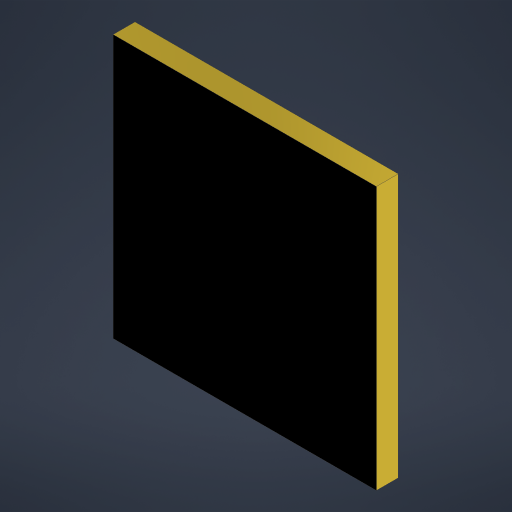
# Autodesk Inventor part: šachovnice
Saved by Autodesk Inventor 2023 (Build 270158000, 158)
## iProperties
Created: 2023-04-20
Part Number: šachovnice
Material: Generic
Document SubType Name: Modeling
Designer: 19LBoreckyP
Density: 1 g/cm^3
Appearance: Wood - Painted White
Author: 19LBoreckyP
Autodesk Inventor part; units mm, degrees
(part 1 of 2)
ref_plane "YZ Plane" through (0, 0, 0) normal (1, 0, 0) x (0, 1, 0)
ref_plane "XZ Plane" through (0, 0, 0) normal (0, 1, 0) x (-1, 0, 0)
ref_plane "XY Plane" through (0, 0, 0) normal (0, 0, 1) x (1, 0, 0)
sketch "Sketch1" plane through (0, 0, 0) normal (0, 0, 1) x (1, 0, 0)
  line L0 (-28.2811, -25.3359) -> (21.7189, -25.3359)
  line L1 (21.7189, -25.3359) -> (21.7189, 24.6641)
  line L2 (21.7189, 24.6641) -> (-28.2811, 24.6641)
  line L3 (-28.2811, 24.6641) -> (-28.2811, -25.3359)
  line L4 (-28.2811, -25.3359) -> (21.7189, 24.6641) construction
  line L5 (21.7189, -25.3359) -> (-28.2811, 24.6641) construction
  line L6 (21.7189, 24.6641) -> (21.7189, 74.6641)
  line L7 (21.7189, 74.6641) -> (-28.2811, 74.6641)
  line L8 (-28.2811, 74.6641) -> (-28.2811, 24.6641)
  line L9 (-28.2811, 24.6641) -> (21.7189, 24.6641)
  line L10 (21.7189, 74.6641) -> (21.7189, 124.6641)
  line L11 (21.7189, 124.6641) -> (-28.2811, 124.6641)
  line L12 (-28.2811, 124.6641) -> (-28.2811, 74.6641)
  line L13 (-28.2811, 74.6641) -> (21.7189, 74.6641)
  line L14 (21.7189, 124.6641) -> (21.7189, 174.6641)
  line L15 (21.7189, 174.6641) -> (-28.2811, 174.6641)
  line L16 (-28.2811, 174.6641) -> (-28.2811, 124.6641)
  line L17 (-28.2811, 124.6641) -> (21.7189, 124.6641)
  line L18 (21.7189, 174.6641) -> (21.7189, 224.6641)
  line L19 (21.7189, 224.6641) -> (-28.2811, 224.6641)
  line L20 (-28.2811, 224.6641) -> (-28.2811, 174.6641)
  line L21 (-28.2811, 174.6641) -> (21.7189, 174.6641)
  line L22 (21.7189, 224.6641) -> (21.7189, 274.6641)
  line L23 (21.7189, 274.6641) -> (-28.2811, 274.6641)
  line L24 (-28.2811, 274.6641) -> (-28.2811, 224.6641)
  line L25 (-28.2811, 224.6641) -> (21.7189, 224.6641)
  line L26 (21.7189, 274.6641) -> (21.7189, 324.6641)
  line L27 (21.7189, 324.6641) -> (-28.2811, 324.6641)
  line L28 (-28.2811, 324.6641) -> (-28.2811, 274.6641)
  line L29 (-28.2811, 274.6641) -> (21.7189, 274.6641)
  line L30 (21.7189, 324.6641) -> (21.7189, 374.6641)
  line L31 (21.7189, 374.6641) -> (-28.2811, 374.6641)
  line L32 (-28.2811, 374.6641) -> (-28.2811, 324.6641)
  line L33 (-28.2811, 324.6641) -> (21.7189, 324.6641)
  line L34 (71.7189, -25.3359) -> (71.7189, 24.6641)
  line L35 (71.7189, 24.6641) -> (21.7189, 24.6641)
  line L36 (21.7189, 24.6641) -> (21.7189, -25.3359)
  line L37 (21.7189, -25.3359) -> (71.7189, -25.3359)
  line L38 (71.7189, 24.6641) -> (71.7189, 74.6641)
  line L39 (71.7189, 74.6641) -> (21.7189, 74.6641)
  line L40 (21.7189, 74.6641) -> (21.7189, 24.6641)
  line L41 (21.7189, 24.6641) -> (71.7189, 24.6641)
  line L42 (71.7189, 74.6641) -> (71.7189, 124.6641)
  line L43 (71.7189, 124.6641) -> (21.7189, 124.6641)
  line L44 (21.7189, 124.6641) -> (21.7189, 74.6641)
  line L45 (21.7189, 74.6641) -> (71.7189, 74.6641)
  line L46 (71.7189, 124.6641) -> (71.7189, 174.6641)
  line L47 (71.7189, 174.6641) -> (21.7189, 174.6641)
  line L48 (21.7189, 174.6641) -> (21.7189, 124.6641)
  line L49 (21.7189, 124.6641) -> (71.7189, 124.6641)
  line L50 (71.7189, 174.6641) -> (71.7189, 224.6641)
  line L51 (71.7189, 224.6641) -> (21.7189, 224.6641)
  line L52 (21.7189, 224.6641) -> (21.7189, 174.6641)
  line L53 (21.7189, 174.6641) -> (71.7189, 174.6641)
  line L54 (71.7189, 224.6641) -> (71.7189, 274.6641)
  line L55 (71.7189, 274.6641) -> (21.7189, 274.6641)
  line L56 (21.7189, 274.6641) -> (21.7189, 224.6641)
  line L57 (21.7189, 224.6641) -> (71.7189, 224.6641)
  line L58 (71.7189, 274.6641) -> (71.7189, 324.6641)
  line L59 (71.7189, 324.6641) -> (21.7189, 324.6641)
  line L60 (21.7189, 324.6641) -> (21.7189, 274.6641)
  line L61 (21.7189, 274.6641) -> (71.7189, 274.6641)
  line L62 (71.7189, 324.6641) -> (71.7189, 374.6641)
  line L63 (71.7189, 374.6641) -> (21.7189, 374.6641)
  line L64 (21.7189, 374.6641) -> (21.7189, 324.6641)
  line L65 (21.7189, 324.6641) -> (71.7189, 324.6641)
  line L66 (121.7189, -25.3359) -> (121.7189, 24.6641)
  line L67 (121.7189, 24.6641) -> (71.7189, 24.6641)
  line L68 (71.7189, 24.6641) -> (71.7189, -25.3359)
  line L69 (71.7189, -25.3359) -> (121.7189, -25.3359)
  line L70 (121.7189, 24.6641) -> (121.7189, 74.6641)
  line L71 (121.7189, 74.6641) -> (71.7189, 74.6641)
  line L72 (71.7189, 74.6641) -> (71.7189, 24.6641)
  line L73 (71.7189, 24.6641) -> (121.7189, 24.6641)
  line L74 (121.7189, 74.6641) -> (121.7189, 124.6641)
  line L75 (121.7189, 124.6641) -> (71.7189, 124.6641)
  line L76 (71.7189, 124.6641) -> (71.7189, 74.6641)
  line L77 (71.7189, 74.6641) -> (121.7189, 74.6641)
  line L78 (121.7189, 124.6641) -> (121.7189, 174.6641)
  line L79 (121.7189, 174.6641) -> (71.7189, 174.6641)
  line L80 (71.7189, 174.6641) -> (71.7189, 124.6641)
  line L81 (71.7189, 124.6641) -> (121.7189, 124.6641)
  line L82 (121.7189, 174.6641) -> (121.7189, 224.6641)
  line L83 (121.7189, 224.6641) -> (71.7189, 224.6641)
  line L84 (71.7189, 224.6641) -> (71.7189, 174.6641)
  line L85 (71.7189, 174.6641) -> (121.7189, 174.6641)
  line L86 (121.7189, 224.6641) -> (121.7189, 274.6641)
  line L87 (121.7189, 274.6641) -> (71.7189, 274.6641)
  line L88 (71.7189, 274.6641) -> (71.7189, 224.6641)
  line L89 (71.7189, 224.6641) -> (121.7189, 224.6641)
  line L90 (121.7189, 274.6641) -> (121.7189, 324.6641)
  line L91 (121.7189, 324.6641) -> (71.7189, 324.6641)
  line L92 (71.7189, 324.6641) -> (71.7189, 274.6641)
  line L93 (71.7189, 274.6641) -> (121.7189, 274.6641)
  line L94 (121.7189, 324.6641) -> (121.7189, 374.6641)
  line L95 (121.7189, 374.6641) -> (71.7189, 374.6641)
  line L96 (71.7189, 374.6641) -> (71.7189, 324.6641)
  line L97 (71.7189, 324.6641) -> (121.7189, 324.6641)
  line L98 (171.7189, -25.3359) -> (171.7189, 24.6641)
  line L99 (171.7189, 24.6641) -> (121.7189, 24.6641)
  line L100 (121.7189, 24.6641) -> (121.7189, -25.3359)
  line L101 (121.7189, -25.3359) -> (171.7189, -25.3359)
  line L102 (171.7189, 24.6641) -> (171.7189, 74.6641)
  line L103 (171.7189, 74.6641) -> (121.7189, 74.6641)
  line L104 (121.7189, 74.6641) -> (121.7189, 24.6641)
  line L105 (121.7189, 24.6641) -> (171.7189, 24.6641)
  line L106 (171.7189, 74.6641) -> (171.7189, 124.6641)
  line L107 (171.7189, 124.6641) -> (121.7189, 124.6641)
  line L108 (121.7189, 124.6641) -> (121.7189, 74.6641)
  line L109 (121.7189, 74.6641) -> (171.7189, 74.6641)
  line L110 (171.7189, 124.6641) -> (171.7189, 174.6641)
  line L111 (171.7189, 174.6641) -> (121.7189, 174.6641)
  line L112 (121.7189, 174.6641) -> (121.7189, 124.6641)
  line L113 (121.7189, 124.6641) -> (171.7189, 124.6641)
  line L114 (171.7189, 174.6641) -> (171.7189, 224.6641)
  line L115 (171.7189, 224.6641) -> (121.7189, 224.6641)
  line L116 (121.7189, 224.6641) -> (121.7189, 174.6641)
  line L117 (121.7189, 174.6641) -> (171.7189, 174.6641)
  line L118 (171.7189, 224.6641) -> (171.7189, 274.6641)
  line L119 (171.7189, 274.6641) -> (121.7189, 274.6641)
  line L120 (121.7189, 274.6641) -> (121.7189, 224.6641)
  line L121 (121.7189, 224.6641) -> (171.7189, 224.6641)
  line L122 (171.7189, 274.6641) -> (171.7189, 324.6641)
  line L123 (171.7189, 324.6641) -> (121.7189, 324.6641)
  line L124 (121.7189, 324.6641) -> (121.7189, 274.6641)
  line L125 (121.7189, 274.6641) -> (171.7189, 274.6641)
  line L126 (171.7189, 324.6641) -> (171.7189, 374.6641)
  line L127 (171.7189, 374.6641) -> (121.7189, 374.6641)
  line L128 (121.7189, 374.6641) -> (121.7189, 324.6641)
  line L129 (121.7189, 324.6641) -> (171.7189, 324.6641)
  line L130 (221.7189, -25.3359) -> (221.7189, 24.6641)
  line L131 (221.7189, 24.6641) -> (171.7189, 24.6641)
  line L132 (171.7189, 24.6641) -> (171.7189, -25.3359)
  line L133 (171.7189, -25.3359) -> (221.7189, -25.3359)
  line L134 (221.7189, 24.6641) -> (221.7189, 74.6641)
  line L135 (221.7189, 74.6641) -> (171.7189, 74.6641)
  line L136 (171.7189, 74.6641) -> (171.7189, 24.6641)
  line L137 (171.7189, 24.6641) -> (221.7189, 24.6641)
  line L138 (221.7189, 74.6641) -> (221.7189, 124.6641)
  line L139 (221.7189, 124.6641) -> (171.7189, 124.6641)
  line L140 (171.7189, 124.6641) -> (171.7189, 74.6641)
  line L141 (171.7189, 74.6641) -> (221.7189, 74.6641)
  line L142 (221.7189, 124.6641) -> (221.7189, 174.6641)
  line L143 (221.7189, 174.6641) -> (171.7189, 174.6641)
  line L144 (171.7189, 174.6641) -> (171.7189, 124.6641)
  line L145 (171.7189, 124.6641) -> (221.7189, 124.6641)
  line L146 (221.7189, 174.6641) -> (221.7189, 224.6641)
  line L147 (221.7189, 224.6641) -> (171.7189, 224.6641)
  line L148 (171.7189, 224.6641) -> (171.7189, 174.6641)
  line L149 (171.7189, 174.6641) -> (221.7189, 174.6641)
  line L150 (221.7189, 224.6641) -> (221.7189, 274.6641)
  line L151 (221.7189, 274.6641) -> (171.7189, 274.6641)
  line L152 (171.7189, 274.6641) -> (171.7189, 224.6641)
  line L153 (171.7189, 224.6641) -> (221.7189, 224.6641)
  line L154 (221.7189, 274.6641) -> (221.7189, 324.6641)
  line L155 (221.7189, 324.6641) -> (171.7189, 324.6641)
  line L156 (171.7189, 324.6641) -> (171.7189, 274.6641)
  line L157 (171.7189, 274.6641) -> (221.7189, 274.6641)
  line L158 (221.7189, 324.6641) -> (221.7189, 374.6641)
  line L159 (221.7189, 374.6641) -> (171.7189, 374.6641)
  line L160 (171.7189, 374.6641) -> (171.7189, 324.6641)
  line L161 (171.7189, 324.6641) -> (221.7189, 324.6641)
  line L162 (271.7189, -25.3359) -> (271.7189, 24.6641)
  line L163 (271.7189, 24.6641) -> (221.7189, 24.6641)
  line L164 (221.7189, 24.6641) -> (221.7189, -25.3359)
  line L165 (221.7189, -25.3359) -> (271.7189, -25.3359)
  line L166 (271.7189, 24.6641) -> (271.7189, 74.6641)
  line L167 (271.7189, 74.6641) -> (221.7189, 74.6641)
  line L168 (221.7189, 74.6641) -> (221.7189, 24.6641)
  line L169 (221.7189, 24.6641) -> (271.7189, 24.6641)
  line L170 (271.7189, 74.6641) -> (271.7189, 124.6641)
  line L171 (271.7189, 124.6641) -> (221.7189, 124.6641)
  line L172 (221.7189, 124.6641) -> (221.7189, 74.6641)
  line L173 (221.7189, 74.6641) -> (271.7189, 74.6641)
  line L174 (271.7189, 124.6641) -> (271.7189, 174.6641)
  line L175 (271.7189, 174.6641) -> (221.7189, 174.6641)
  line L176 (221.7189, 174.6641) -> (221.7189, 124.6641)
  line L177 (221.7189, 124.6641) -> (271.7189, 124.6641)
  line L178 (271.7189, 174.6641) -> (271.7189, 224.6641)
  line L179 (271.7189, 224.6641) -> (221.7189, 224.6641)
  line L180 (221.7189, 224.6641) -> (221.7189, 174.6641)
  line L181 (221.7189, 174.6641) -> (271.7189, 174.6641)
  line L182 (271.7189, 224.6641) -> (271.7189, 274.6641)
  line L183 (271.7189, 274.6641) -> (221.7189, 274.6641)
  line L184 (221.7189, 274.6641) -> (221.7189, 224.6641)
  line L185 (221.7189, 224.6641) -> (271.7189, 224.6641)
  line L186 (271.7189, 274.6641) -> (271.7189, 324.6641)
  line L187 (271.7189, 324.6641) -> (221.7189, 324.6641)
  line L188 (221.7189, 324.6641) -> (221.7189, 274.6641)
  line L189 (221.7189, 274.6641) -> (271.7189, 274.6641)
  line L190 (271.7189, 324.6641) -> (271.7189, 374.6641)
  line L191 (271.7189, 374.6641) -> (221.7189, 374.6641)
  line L192 (221.7189, 374.6641) -> (221.7189, 324.6641)
  line L193 (221.7189, 324.6641) -> (271.7189, 324.6641)
  line L194 (321.7189, -25.3359) -> (321.7189, 24.6641)
  line L195 (321.7189, 24.6641) -> (271.7189, 24.6641)
  line L196 (271.7189, 24.6641) -> (271.7189, -25.3359)
  line L197 (271.7189, -25.3359) -> (321.7189, -25.3359)
  line L198 (321.7189, 24.6641) -> (321.7189, 74.6641)
  line L199 (321.7189, 74.6641) -> (271.7189, 74.6641)
  line L200 (271.7189, 74.6641) -> (271.7189, 24.6641)
  line L201 (271.7189, 24.6641) -> (321.7189, 24.6641)
  line L202 (321.7189, 74.6641) -> (321.7189, 124.6641)
  line L203 (321.7189, 124.6641) -> (271.7189, 124.6641)
  line L204 (271.7189, 124.6641) -> (271.7189, 74.6641)
  line L205 (271.7189, 74.6641) -> (321.7189, 74.6641)
  line L206 (321.7189, 124.6641) -> (321.7189, 174.6641)
  line L207 (321.7189, 174.6641) -> (271.7189, 174.6641)
  line L208 (271.7189, 174.6641) -> (271.7189, 124.6641)
  line L209 (271.7189, 124.6641) -> (321.7189, 124.6641)
  line L210 (321.7189, 174.6641) -> (321.7189, 224.6641)
  line L211 (321.7189, 224.6641) -> (271.7189, 224.6641)
  line L212 (271.7189, 224.6641) -> (271.7189, 174.6641)
  line L213 (271.7189, 174.6641) -> (321.7189, 174.6641)
  line L214 (321.7189, 224.6641) -> (321.7189, 274.6641)
  line L215 (321.7189, 274.6641) -> (271.7189, 274.6641)
  line L216 (271.7189, 274.6641) -> (271.7189, 224.6641)
  line L217 (271.7189, 224.6641) -> (321.7189, 224.6641)
  line L218 (321.7189, 274.6641) -> (321.7189, 324.6641)
  line L219 (321.7189, 324.6641) -> (271.7189, 324.6641)
  line L220 (271.7189, 324.6641) -> (271.7189, 274.6641)
  line L221 (271.7189, 274.6641) -> (321.7189, 274.6641)
  line L222 (321.7189, 324.6641) -> (321.7189, 374.6641)
  line L223 (321.7189, 374.6641) -> (271.7189, 374.6641)
  line L224 (271.7189, 374.6641) -> (271.7189, 324.6641)
  line L225 (271.7189, 324.6641) -> (321.7189, 324.6641)
  line L226 (371.7189, -25.3359) -> (371.7189, 24.6641)
  line L227 (371.7189, 24.6641) -> (321.7189, 24.6641)
  line L228 (321.7189, 24.6641) -> (321.7189, -25.3359)
  line L229 (321.7189, -25.3359) -> (371.7189, -25.3359)
  line L230 (371.7189, 24.6641) -> (371.7189, 74.6641)
  line L231 (371.7189, 74.6641) -> (321.7189, 74.6641)
  line L232 (321.7189, 74.6641) -> (321.7189, 24.6641)
  line L233 (321.7189, 24.6641) -> (371.7189, 24.6641)
  line L234 (371.7189, 74.6641) -> (371.7189, 124.6641)
  line L235 (371.7189, 124.6641) -> (321.7189, 124.6641)
  line L236 (321.7189, 124.6641) -> (321.7189, 74.6641)
  line L237 (321.7189, 74.6641) -> (371.7189, 74.6641)
  line L238 (371.7189, 124.6641) -> (371.7189, 174.6641)
  line L239 (371.7189, 174.6641) -> (321.7189, 174.6641)
  line L240 (321.7189, 174.6641) -> (321.7189, 124.6641)
  line L241 (321.7189, 124.6641) -> (371.7189, 124.6641)
  line L242 (371.7189, 174.6641) -> (371.7189, 224.6641)
  line L243 (371.7189, 224.6641) -> (321.7189, 224.6641)
  line L244 (321.7189, 224.6641) -> (321.7189, 174.6641)
  line L245 (321.7189, 174.6641) -> (371.7189, 174.6641)
  line L246 (371.7189, 224.6641) -> (371.7189, 274.6641)
  line L247 (371.7189, 274.6641) -> (321.7189, 274.6641)
  line L248 (321.7189, 274.6641) -> (321.7189, 224.6641)
  line L249 (321.7189, 224.6641) -> (371.7189, 224.6641)
  line L250 (371.7189, 274.6641) -> (371.7189, 324.6641)
  line L251 (371.7189, 324.6641) -> (321.7189, 324.6641)
  line L252 (321.7189, 324.6641) -> (321.7189, 274.6641)
  line L253 (321.7189, 274.6641) -> (371.7189, 274.6641)
  line L254 (371.7189, 324.6641) -> (371.7189, 374.6641)
  line L255 (371.7189, 374.6641) -> (321.7189, 374.6641)
  line L256 (321.7189, 374.6641) -> (321.7189, 324.6641)
  line L257 (321.7189, 324.6641) -> (371.7189, 324.6641)
  point P0 (0, 0)
  point P1 (-3.2811, -0.3359)
  point P2 (-28.2811, 274.6641)
  point P3 (-28.2811, 174.6641)
  point P4 (-28.2811, 74.6641)
  dimension "d0" = 50
  dimension "d1" = 50
  dimension "d4" = 50
  dimension "d7" = 50
  constraints: 516 end point, 2 collinear, 2 horizontal, 2 midpoint, 2 parallel, 1 perpendicular, 1 vertical, 502 other
  measures "d0" distance of L2.end L1.end
  measures "d1" distance of L1.end L0.end
  measures "d4" distance of L0.end L6.start
  measures "d7" distance of L0.end L34.start
extrude "Extrusion1" add sketch "Sketch1" along normal blind 1 contours L3 L2 L1 L0 | L6 L39 L38 L35 | L34 L67 L66 L69 | L12 L11 L10 L7 | L14 L47 L46 L43 | L42 L75 L74 L71 | L70 L103 L102 L99 | L98 L131 L130 L133 | L20 L19 L18 L15 | L22 L55 L54 L51 | L50 L83 L82 L79 | L78 L111 L110 L107 | L106 L139 L138 L135 | L134 L167 L166 L163 | L162 L195 L194 L197 | L28 L27 L26 L23 | L30 L63 L62 L59 | L58 L91 L90 L87 | L86 L119 L118 L115 | L114 L147 L146 L143 | L142 L175 L174 L171 | L170 L203 L202 L199 | L198 L231 L230 L227 | L94 L127 L126 L123 | L122 L155 L154 L151 | L150 L183 L182 L179 | L178 L211 L210 L207 | L206 L239 L238 L235 | L158 L191 L190 L187 | L186 L219 L218 L215 | L214 L247 L246 L243 | L222 L255 L254 L251
sketch "Sketch2" plane through (0, 0, 1) normal (0, 0, 1) x (1, 0, 0)
  line L0 (-28.2811, -25.3359) -> (21.7189, -25.3359) projected
  line L1 (21.7189, -25.3359) -> (21.7189, 24.6641) projected
  line L2 (21.7189, 24.6641) -> (-28.2811, 24.6641) projected
  line L3 (-28.2811, 24.6641) -> (-28.2811, -25.3359) projected
  line L4 (-28.2811, 24.6641) -> (-28.2811, -25.3359) projected
  line L5 (-28.2811, 24.6641) -> (-28.2811, -25.3359)
  line L6 (-28.2811, -25.3359) -> (21.7189, -25.3359) projected
  line L7 (-28.2811, -25.3359) -> (21.7189, -25.3359)
  line L8 (21.7189, -25.3359) -> (21.7189, 24.6641) projected
  line L9 (21.7189, -25.3359) -> (21.7189, 24.6641)
  line L10 (21.7189, 24.6641) -> (-28.2811, 24.6641) projected
  line L11 (21.7189, 24.6641) -> (-28.2811, 24.6641)
  line L12 (21.7189, 74.6641) -> (-28.2811, 74.6641)
  line L13 (21.7189, 24.6641) -> (21.7189, 74.6641)
  line L14 (-28.2811, 24.6641) -> (21.7189, 24.6641)
  line L15 (-28.2811, 74.6641) -> (-28.2811, 24.6641)
  line L16 (21.7189, 124.6641) -> (-28.2811, 124.6641)
  line L17 (21.7189, 74.6641) -> (21.7189, 124.6641)
  line L18 (-28.2811, 74.6641) -> (21.7189, 74.6641)
  line L19 (-28.2811, 124.6641) -> (-28.2811, 74.6641)
  line L20 (21.7189, 174.6641) -> (-28.2811, 174.6641)
  line L21 (21.7189, 124.6641) -> (21.7189, 174.6641)
  line L22 (-28.2811, 124.6641) -> (21.7189, 124.6641)
  line L23 (-28.2811, 174.6641) -> (-28.2811, 124.6641)
  line L24 (21.7189, 224.6641) -> (-28.2811, 224.6641)
  line L25 (21.7189, 174.6641) -> (21.7189, 224.6641)
  line L26 (-28.2811, 174.6641) -> (21.7189, 174.6641)
  line L27 (-28.2811, 224.6641) -> (-28.2811, 174.6641)
  line L28 (21.7189, 274.6641) -> (-28.2811, 274.6641)
  line L29 (21.7189, 224.6641) -> (21.7189, 274.6641)
  line L30 (-28.2811, 224.6641) -> (21.7189, 224.6641)
  line L31 (-28.2811, 274.6641) -> (-28.2811, 224.6641)
  line L32 (21.7189, 324.6641) -> (-28.2811, 324.6641)
  line L33 (21.7189, 274.6641) -> (21.7189, 324.6641)
  line L34 (-28.2811, 274.6641) -> (21.7189, 274.6641)
  line L35 (-28.2811, 324.6641) -> (-28.2811, 274.6641)
  line L36 (21.7189, 374.6641) -> (-28.2811, 374.6641)
  line L37 (21.7189, 324.6641) -> (21.7189, 374.6641)
  line L38 (-28.2811, 324.6641) -> (21.7189, 324.6641)
  line L39 (-28.2811, 374.6641) -> (-28.2811, 324.6641)
  line L40 (71.7189, 24.6641) -> (21.7189, 24.6641)
  line L41 (71.7189, -25.3359) -> (71.7189, 24.6641)
  line L42 (21.7189, -25.3359) -> (71.7189, -25.3359)
  line L43 (21.7189, 24.6641) -> (21.7189, -25.3359)
  line L44 (71.7189, 74.6641) -> (21.7189, 74.6641)
  line L45 (71.7189, 24.6641) -> (71.7189, 74.6641)
  line L46 (21.7189, 24.6641) -> (71.7189, 24.6641)
  line L47 (21.7189, 74.6641) -> (21.7189, 24.6641)
  line L48 (71.7189, 124.6641) -> (21.7189, 124.6641)
  line L49 (71.7189, 74.6641) -> (71.7189, 124.6641)
  line L50 (21.7189, 74.6641) -> (71.7189, 74.6641)
  line L51 (21.7189, 124.6641) -> (21.7189, 74.6641)
  line L52 (71.7189, 174.6641) -> (21.7189, 174.6641)
  line L53 (71.7189, 124.6641) -> (71.7189, 174.6641)
  line L54 (21.7189, 124.6641) -> (71.7189, 124.6641)
  line L55 (21.7189, 174.6641) -> (21.7189, 124.6641)
  line L56 (71.7189, 224.6641) -> (21.7189, 224.6641)
  line L57 (71.7189, 174.6641) -> (71.7189, 224.6641)
  line L58 (21.7189, 174.6641) -> (71.7189, 174.6641)
  line L59 (21.7189, 224.6641) -> (21.7189, 174.6641)
  line L60 (71.7189, 274.6641) -> (21.7189, 274.6641)
  line L61 (71.7189, 224.6641) -> (71.7189, 274.6641)
  line L62 (21.7189, 224.6641) -> (71.7189, 224.6641)
  line L63 (21.7189, 274.6641) -> (21.7189, 224.6641)
  line L64 (71.7189, 324.6641) -> (21.7189, 324.6641)
  line L65 (71.7189, 274.6641) -> (71.7189, 324.6641)
  line L66 (21.7189, 274.6641) -> (71.7189, 274.6641)
  line L67 (21.7189, 324.6641) -> (21.7189, 274.6641)
  line L68 (71.7189, 374.6641) -> (21.7189, 374.6641)
  line L69 (71.7189, 324.6641) -> (71.7189, 374.6641)
  line L70 (21.7189, 324.6641) -> (71.7189, 324.6641)
  line L71 (21.7189, 374.6641) -> (21.7189, 324.6641)
  line L72 (121.7189, 24.6641) -> (71.7189, 24.6641)
  line L73 (121.7189, -25.3359) -> (121.7189, 24.6641)
  line L74 (71.7189, -25.3359) -> (121.7189, -25.3359)
  line L75 (71.7189, 24.6641) -> (71.7189, -25.3359)
  line L76 (121.7189, 74.6641) -> (71.7189, 74.6641)
  line L77 (121.7189, 24.6641) -> (121.7189, 74.6641)
  line L78 (71.7189, 24.6641) -> (121.7189, 24.6641)
  line L79 (71.7189, 74.6641) -> (71.7189, 24.6641)
  line L80 (121.7189, 124.6641) -> (71.7189, 124.6641)
  line L81 (121.7189, 74.6641) -> (121.7189, 124.6641)
  line L82 (71.7189, 74.6641) -> (121.7189, 74.6641)
  line L83 (71.7189, 124.6641) -> (71.7189, 74.6641)
  line L84 (121.7189, 174.6641) -> (71.7189, 174.6641)
  line L85 (121.7189, 124.6641) -> (121.7189, 174.6641)
  line L86 (71.7189, 124.6641) -> (121.7189, 124.6641)
  line L87 (71.7189, 174.6641) -> (71.7189, 124.6641)
  line L88 (121.7189, 224.6641) -> (71.7189, 224.6641)
  line L89 (121.7189, 174.6641) -> (121.7189, 224.6641)
  line L90 (71.7189, 174.6641) -> (121.7189, 174.6641)
  line L91 (71.7189, 224.6641) -> (71.7189, 174.6641)
  line L92 (121.7189, 274.6641) -> (71.7189, 274.6641)
  line L93 (121.7189, 224.6641) -> (121.7189, 274.6641)
  line L94 (71.7189, 224.6641) -> (121.7189, 224.6641)
  line L95 (71.7189, 274.6641) -> (71.7189, 224.6641)
  line L96 (121.7189, 324.6641) -> (71.7189, 324.6641)
  line L97 (121.7189, 274.6641) -> (121.7189, 324.6641)
  line L98 (71.7189, 274.6641) -> (121.7189, 274.6641)
  line L99 (71.7189, 324.6641) -> (71.7189, 274.6641)
  line L100 (121.7189, 374.6641) -> (71.7189, 374.6641)
  line L101 (121.7189, 324.6641) -> (121.7189, 374.6641)
  line L102 (71.7189, 324.6641) -> (121.7189, 324.6641)
  line L103 (71.7189, 374.6641) -> (71.7189, 324.6641)
  line L104 (171.7189, 24.6641) -> (121.7189, 24.6641)
  line L105 (171.7189, -25.3359) -> (171.7189, 24.6641)
  line L106 (121.7189, -25.3359) -> (171.7189, -25.3359)
  line L107 (121.7189, 24.6641) -> (121.7189, -25.3359)
  line L108 (171.7189, 74.6641) -> (121.7189, 74.6641)
  line L109 (171.7189, 24.6641) -> (171.7189, 74.6641)
  line L110 (121.7189, 24.6641) -> (171.7189, 24.6641)
  line L111 (121.7189, 74.6641) -> (121.7189, 24.6641)
  line L112 (171.7189, 124.6641) -> (121.7189, 124.6641)
  line L113 (171.7189, 74.6641) -> (171.7189, 124.6641)
  line L114 (121.7189, 74.6641) -> (171.7189, 74.6641)
  line L115 (121.7189, 124.6641) -> (121.7189, 74.6641)
  line L116 (171.7189, 174.6641) -> (121.7189, 174.6641)
  line L117 (171.7189, 124.6641) -> (171.7189, 174.6641)
  line L118 (121.7189, 124.6641) -> (171.7189, 124.6641)
  line L119 (121.7189, 174.6641) -> (121.7189, 124.6641)
  line L120 (171.7189, 224.6641) -> (121.7189, 224.6641)
  line L121 (171.7189, 174.6641) -> (171.7189, 224.6641)
  line L122 (121.7189, 174.6641) -> (171.7189, 174.6641)
  line L123 (121.7189, 224.6641) -> (121.7189, 174.6641)
  line L124 (171.7189, 274.6641) -> (121.7189, 274.6641)
  line L125 (171.7189, 224.6641) -> (171.7189, 274.6641)
  line L126 (121.7189, 224.6641) -> (171.7189, 224.6641)
  line L127 (121.7189, 274.6641) -> (121.7189, 224.6641)
  line L128 (171.7189, 324.6641) -> (121.7189, 324.6641)
  line L129 (171.7189, 274.6641) -> (171.7189, 324.6641)
  line L130 (121.7189, 274.6641) -> (171.7189, 274.6641)
  line L131 (121.7189, 324.6641) -> (121.7189, 274.6641)
  line L132 (171.7189, 374.6641) -> (121.7189, 374.6641)
  line L133 (171.7189, 324.6641) -> (171.7189, 374.6641)
  line L134 (121.7189, 324.6641) -> (171.7189, 324.6641)
  line L135 (121.7189, 374.6641) -> (121.7189, 324.6641)
  line L136 (221.7189, 24.6641) -> (171.7189, 24.6641)
  line L137 (221.7189, -25.3359) -> (221.7189, 24.6641)
  line L138 (171.7189, -25.3359) -> (221.7189, -25.3359)
  line L139 (171.7189, 24.6641) -> (171.7189, -25.3359)
  line L140 (221.7189, 74.6641) -> (171.7189, 74.6641)
  line L141 (221.7189, 24.6641) -> (221.7189, 74.6641)
  line L142 (171.7189, 24.6641) -> (221.7189, 24.6641)
  line L143 (171.7189, 74.6641) -> (171.7189, 24.6641)
  line L144 (221.7189, 124.6641) -> (171.7189, 124.6641)
  line L145 (221.7189, 74.6641) -> (221.7189, 124.6641)
  line L146 (171.7189, 74.6641) -> (221.7189, 74.6641)
  line L147 (171.7189, 124.6641) -> (171.7189, 74.6641)
  line L148 (221.7189, 174.6641) -> (171.7189, 174.6641)
  line L149 (221.7189, 124.6641) -> (221.7189, 174.6641)
  line L150 (171.7189, 124.6641) -> (221.7189, 124.6641)
  line L151 (171.7189, 174.6641) -> (171.7189, 124.6641)
  line L152 (221.7189, 224.6641) -> (171.7189, 224.6641)
  line L153 (221.7189, 174.6641) -> (221.7189, 224.6641)
  line L154 (171.7189, 174.6641) -> (221.7189, 174.6641)
  line L155 (171.7189, 224.6641) -> (171.7189, 174.6641)
  line L156 (221.7189, 274.6641) -> (171.7189, 274.6641)
  line L157 (221.7189, 224.6641) -> (221.7189, 274.6641)
  line L158 (171.7189, 224.6641) -> (221.7189, 224.6641)
  line L159 (171.7189, 274.6641) -> (171.7189, 224.6641)
  line L160 (221.7189, 324.6641) -> (171.7189, 324.6641)
  line L161 (221.7189, 274.6641) -> (221.7189, 324.6641)
  line L162 (171.7189, 274.6641) -> (221.7189, 274.6641)
  line L163 (171.7189, 324.6641) -> (171.7189, 274.6641)
  line L164 (221.7189, 374.6641) -> (171.7189, 374.6641)
  line L165 (221.7189, 324.6641) -> (221.7189, 374.6641)
  line L166 (171.7189, 324.6641) -> (221.7189, 324.6641)
  line L167 (171.7189, 374.6641) -> (171.7189, 324.6641)
  line L168 (271.7189, 24.6641) -> (221.7189, 24.6641)
  line L169 (271.7189, -25.3359) -> (271.7189, 24.6641)
  line L170 (221.7189, -25.3359) -> (271.7189, -25.3359)
  line L171 (221.7189, 24.6641) -> (221.7189, -25.3359)
  line L172 (271.7189, 74.6641) -> (221.7189, 74.6641)
  line L173 (271.7189, 24.6641) -> (271.7189, 74.6641)
  line L174 (221.7189, 24.6641) -> (271.7189, 24.6641)
  line L175 (221.7189, 74.6641) -> (221.7189, 24.6641)
  line L176 (271.7189, 124.6641) -> (221.7189, 124.6641)
  line L177 (271.7189, 74.6641) -> (271.7189, 124.6641)
  line L178 (221.7189, 74.6641) -> (271.7189, 74.6641)
  line L179 (221.7189, 124.6641) -> (221.7189, 74.6641)
  line L180 (271.7189, 174.6641) -> (221.7189, 174.6641)
  line L181 (271.7189, 124.6641) -> (271.7189, 174.6641)
  line L182 (221.7189, 124.6641) -> (271.7189, 124.6641)
  line L183 (221.7189, 174.6641) -> (221.7189, 124.6641)
  line L184 (271.7189, 224.6641) -> (221.7189, 224.6641)
  line L185 (271.7189, 174.6641) -> (271.7189, 224.6641)
  line L186 (221.7189, 174.6641) -> (271.7189, 174.6641)
  line L187 (221.7189, 224.6641) -> (221.7189, 174.6641)
  line L188 (271.7189, 274.6641) -> (221.7189, 274.6641)
  line L189 (271.7189, 224.6641) -> (271.7189, 274.6641)
  line L190 (221.7189, 224.6641) -> (271.7189, 224.6641)
  line L191 (221.7189, 274.6641) -> (221.7189, 224.6641)
  line L192 (271.7189, 324.6641) -> (221.7189, 324.6641)
  line L193 (271.7189, 274.6641) -> (271.7189, 324.6641)
  line L194 (221.7189, 274.6641) -> (271.7189, 274.6641)
  line L195 (221.7189, 324.6641) -> (221.7189, 274.6641)
  line L196 (271.7189, 374.6641) -> (221.7189, 374.6641)
  line L197 (271.7189, 324.6641) -> (271.7189, 374.6641)
  line L198 (221.7189, 324.6641) -> (271.7189, 324.6641)
  line L199 (221.7189, 374.6641) -> (221.7189, 324.6641)
  line L200 (321.7189, 24.6641) -> (271.7189, 24.6641)
  line L201 (321.7189, -25.3359) -> (321.7189, 24.6641)
  line L202 (271.7189, -25.3359) -> (321.7189, -25.3359)
  line L203 (271.7189, 24.6641) -> (271.7189, -25.3359)
  line L204 (321.7189, 74.6641) -> (271.7189, 74.6641)
  line L205 (321.7189, 24.6641) -> (321.7189, 74.6641)
  line L206 (271.7189, 24.6641) -> (321.7189, 24.6641)
  line L207 (271.7189, 74.6641) -> (271.7189, 24.6641)
  line L208 (321.7189, 124.6641) -> (271.7189, 124.6641)
  line L209 (321.7189, 74.6641) -> (321.7189, 124.6641)
  line L210 (271.7189, 74.6641) -> (321.7189, 74.6641)
  line L211 (271.7189, 124.6641) -> (271.7189, 74.6641)
  line L212 (321.7189, 174.6641) -> (271.7189, 174.6641)
  line L213 (321.7189, 124.6641) -> (321.7189, 174.6641)
  line L214 (271.7189, 124.6641) -> (321.7189, 124.6641)
  line L215 (271.7189, 174.6641) -> (271.7189, 124.6641)
  line L216 (321.7189, 224.6641) -> (271.7189, 224.6641)
  line L217 (321.7189, 174.6641) -> (321.7189, 224.6641)
  line L218 (271.7189, 174.6641) -> (321.7189, 174.6641)
  line L219 (271.7189, 224.6641) -> (271.7189, 174.6641)
  line L220 (321.7189, 274.6641) -> (271.7189, 274.6641)
  line L221 (321.7189, 224.6641) -> (321.7189, 274.6641)
  line L222 (271.7189, 224.6641) -> (321.7189, 224.6641)
  line L223 (271.7189, 274.6641) -> (271.7189, 224.6641)
  line L224 (321.7189, 324.6641) -> (271.7189, 324.6641)
  line L225 (321.7189, 274.6641) -> (321.7189, 324.6641)
  line L226 (271.7189, 274.6641) -> (321.7189, 274.6641)
  line L227 (271.7189, 324.6641) -> (271.7189, 274.6641)
  line L228 (321.7189, 374.6641) -> (271.7189, 374.6641)
  line L229 (321.7189, 324.6641) -> (321.7189, 374.6641)
  line L230 (271.7189, 324.6641) -> (321.7189, 324.6641)
  line L231 (271.7189, 374.6641) -> (271.7189, 324.6641)
  line L232 (371.7189, 24.6641) -> (321.7189, 24.6641)
  line L233 (371.7189, -25.3359) -> (371.7189, 24.6641)
  line L234 (321.7189, -25.3359) -> (371.7189, -25.3359)
  line L235 (321.7189, 24.6641) -> (321.7189, -25.3359)
  line L236 (371.7189, 74.6641) -> (321.7189, 74.6641)
  line L237 (371.7189, 24.6641) -> (371.7189, 74.6641)
  line L238 (321.7189, 24.6641) -> (371.7189, 24.6641)
  line L239 (321.7189, 74.6641) -> (321.7189, 24.6641)
  line L240 (371.7189, 124.6641) -> (321.7189, 124.6641)
  line L241 (371.7189, 74.6641) -> (371.7189, 124.6641)
  line L242 (321.7189, 74.6641) -> (371.7189, 74.6641)
  line L243 (321.7189, 124.6641) -> (321.7189, 74.6641)
  line L244 (371.7189, 174.6641) -> (321.7189, 174.6641)
  line L245 (371.7189, 124.6641) -> (371.7189, 174.6641)
  line L246 (321.7189, 124.6641) -> (371.7189, 124.6641)
  line L247 (321.7189, 174.6641) -> (321.7189, 124.6641)
  line L248 (371.7189, 224.6641) -> (321.7189, 224.6641)
  line L249 (371.7189, 174.6641) -> (371.7189, 224.6641)
  line L250 (321.7189, 174.6641) -> (371.7189, 174.6641)
  line L251 (321.7189, 224.6641) -> (321.7189, 174.6641)
  line L252 (371.7189, 274.6641) -> (321.7189, 274.6641)
  line L253 (371.7189, 224.6641) -> (371.7189, 274.6641)
  line L254 (321.7189, 224.6641) -> (371.7189, 224.6641)
  line L255 (321.7189, 274.6641) -> (321.7189, 224.6641)
  line L256 (371.7189, 324.6641) -> (321.7189, 324.6641)
  line L257 (371.7189, 274.6641) -> (371.7189, 324.6641)
  line L258 (321.7189, 274.6641) -> (371.7189, 274.6641)
  line L259 (321.7189, 324.6641) -> (321.7189, 274.6641)
  line L260 (371.7189, 374.6641) -> (321.7189, 374.6641)
  line L261 (371.7189, 324.6641) -> (371.7189, 374.6641)
  line L262 (321.7189, 324.6641) -> (371.7189, 324.6641)
  line L263 (321.7189, 374.6641) -> (321.7189, 324.6641)
  point P0 (0, 0)
  dimension "d14" = 50
  dimension "d17" = 50
  constraints: 512 end point, 2 collinear, 2 vertical, 1 horizontal, 1 perpendicular, 504 other
  measures "d14" distance of L1.end L12.start
  measures "d17" distance of L1.end L40.start
extrude "Extrusion2" add sketch "Sketch2" against normal blind 0.99 contours L1 L40 L41 L42 | L15 L12 L13 L2 | L17 L48 L49 L44 | L45 L76 L77 L72 | L73 L104 L105 L106 | L23 L20 L21 L16 | L25 L56 L57 L52 | L53 L84 L85 L80 | L81 L112 L113 L108 | L109 L140 L141 L136 | L137 L168 L169 L170 | L31 L28 L29 L24 | L33 L64 L65 L60 | L61 L92 L93 L88 | L89 L120 L121 L116 | L117 L148 L149 L144 | L145 L176 L177 L172 | L173 L204 L205 L200 | L201 L232 L233 L234 | L39 L36 L37 L32 | L69 L100 L101 L96 | L97 L128 L129 L124 | L125 L156 L157 L152 | L153 L184 L185 L180 | L181 L212 L213 L208 | L209 L240 L241 L236 | L133 L164 L165 L160 | L161 L192 L193 L188 | L189 L220 L221 L216 | L217 L248 L249 L244 | L197 L228 L229 L224 | L225 L256 L257 L252
sketch "Sketch5" plane through (21.7189, 374.6641, 0) normal (0, 1, 0) x (1, 0, 0)
  point P0 (-21.7189, 0)
sketch "Sketch6" plane through (0, 0, 1) normal (0, 0, 1) x (1, 0, 0)
  line L0 (-28.2811, 374.6641) -> (-28.2811, -25.3359) projected
  line L1 (-28.2811, -25.3359) -> (-38.8877, -35.9425)
  line L2 (-28.2811, -25.3359) -> (-13.2811, -25.3359) construction
  line L3 (371.7189, 374.6641) -> (382.3255, 385.2707)
  line L4 (-38.8877, -35.9425) -> (382.3255, -35.9425)
  line L5 (382.3255, -35.9425) -> (382.3255, 385.2707)
  line L6 (382.3255, 385.2707) -> (-38.8877, 385.2707)
  line L7 (-38.8877, 385.2707) -> (-38.8877, -35.9425)
  point P0 (0, 0)
  dimension "d26" = 15
  dimension "d27" = 135
  dimension "d28" = 15
  constraints: 14 end point, 2 horizontal, 2 parallel, 1 equal length, 1 perpendicular
  measures "d26" distance of L0.end L1.end
  measures "d27" angle of L1 L2
  measures "d28" distance of L3.start L3.end
extrude "Extrusion3" add sketch "Sketch6" along normal blind 35
sketch "Sketch7" plane through (0, 0, 1) normal (0, 0, -1) x (-1, 0, 0)
  line L0 (38.8877, -33.4425) -> (-382.3255, -33.4425) construction
  line L1 (-371.7189, 24.6641) -> (-321.7189, 24.6641) projected
  line L2 (-371.7189, 24.6641) -> (-371.7189, -25.3359) projected
  line L3 (-371.7189, -25.3359) -> (-321.7189, -25.3359) projected
  line L4 (-321.7189, 24.6641) -> (-321.7189, -25.3359) projected
  line L5 (-321.7189, -25.3359) -> (-321.7189, 24.6641) projected
  line L6 (-271.7189, -25.3359) -> (-321.7189, -25.3359) projected
  line L7 (-271.7189, 24.6641) -> (-271.7189, -25.3359) projected
  line L8 (-321.7189, 24.6641) -> (-271.7189, 24.6641) projected
  line L9 (-271.7189, -25.3359) -> (-271.7189, 24.6641) projected
  line L10 (-271.7189, -25.3359) -> (-221.7189, -25.3359) projected
  line L11 (-221.7189, 24.6641) -> (-221.7189, -25.3359) projected
  line L12 (-271.7189, 24.6641) -> (-221.7189, 24.6641) projected
  line L13 (-221.7189, -25.3359) -> (-221.7189, 24.6641) projected
  line L14 (-171.7189, -25.3359) -> (-221.7189, -25.3359) projected
  line L15 (-171.7189, 24.6641) -> (-171.7189, -25.3359) projected
  line L16 (-221.7189, 24.6641) -> (-171.7189, 24.6641) projected
  line L17 (-171.7189, -25.3359) -> (-171.7189, 24.6641) projected
  line L18 (-171.7189, -25.3359) -> (-121.7189, -25.3359) projected
  line L19 (-121.7189, 24.6641) -> (-121.7189, -25.3359) projected
  line L20 (-171.7189, 24.6641) -> (-121.7189, 24.6641) projected
  line L21 (-121.7189, -25.3359) -> (-121.7189, 24.6641) projected
  line L22 (-71.7189, -25.3359) -> (-121.7189, -25.3359) projected
  line L23 (-71.7189, 24.6641) -> (-71.7189, -25.3359) projected
  line L24 (-121.7189, 24.6641) -> (-71.7189, 24.6641) projected
  line L25 (-71.7189, -25.3359) -> (-71.7189, 24.6641) projected
  line L26 (-71.7189, -25.3359) -> (-21.7189, -25.3359) projected
  line L27 (-21.7189, 24.6641) -> (-21.7189, -25.3359) projected
  line L28 (-71.7189, 24.6641) -> (-21.7189, 24.6641) projected
  line L29 (28.2811, -25.3359) -> (-21.7189, -25.3359) projected
  line L30 (28.2811, 24.6641) -> (28.2811, -25.3359) projected
  line L31 (-21.7189, 24.6641) -> (28.2811, 24.6641) projected
  line L32 (-21.7189, -25.3359) -> (-21.7189, 24.6641) projected
  line L33 (-371.7189, -25.3359) -> (-321.7189, -25.3359) projected
  line L34 (-350.4742, -27.4339) -> (-342.9636, -27.4339) construction
  line L35 (-342.9636, -27.4339) -> (-342.9636, -33.4425) construction
  line L36 (-342.9636, -33.4425) -> (-350.4742, -33.4425) construction
  line L37 (-350.4742, -33.4425) -> (-350.4742, -27.4339) construction
  line L38 (-304.4799, -26.5994) -> (-288.9579, -26.5994) construction
  line L39 (-288.9579, -26.5994) -> (-288.9579, -33.4425) construction
  line L40 (-288.9579, -33.4425) -> (-304.4799, -33.4425) construction
  line L41 (-304.4799, -33.4425) -> (-304.4799, -26.5994) construction
  line L42 (-255.5584, -27.1286) -> (-237.8794, -27.1286) construction
  line L43 (-237.8794, -27.1286) -> (-237.8794, -33.4425) construction
  line L44 (-237.8794, -33.4425) -> (-255.5584, -33.4425) construction
  line L45 (-255.5584, -33.4425) -> (-255.5584, -27.1286) construction
  line L46 (-204.927, -26.3709) -> (-188.5108, -26.3709) construction
  line L47 (-188.5108, -26.3709) -> (-188.5108, -33.4425) construction
  line L48 (-188.5108, -33.4425) -> (-204.927, -33.4425) construction
  line L49 (-204.927, -33.4425) -> (-204.927, -26.3709) construction
  line L50 (-156.1898, -25.8658) -> (-137.248, -25.8658) construction
  line L51 (-137.248, -25.8658) -> (-137.248, -33.4425) construction
  line L52 (-137.248, -33.4425) -> (-156.1898, -33.4425) construction
  line L53 (-156.1898, -33.4425) -> (-156.1898, -25.8658) construction
  line L54 (-107.3263, -25.1081) -> (-86.1115, -25.1081) construction
  line L55 (-86.1115, -25.1081) -> (-86.1115, -33.4425) construction
  line L56 (-86.1115, -33.4425) -> (-107.3263, -33.4425) construction
  line L57 (-107.3263, -33.4425) -> (-107.3263, -25.1081) construction
  line L58 (-57.4525, -25.1081) -> (-35.9853, -25.1081) construction
  line L59 (-35.9853, -25.1081) -> (-35.9853, -33.4425) construction
  line L60 (-35.9853, -33.4425) -> (-57.4525, -33.4425) construction
  line L61 (-57.4525, -33.4425) -> (-57.4525, -25.1081) construction
  line L62 (-9.9781, -25.3607) -> (16.5403, -25.3607) construction
  line L63 (16.5403, -25.3607) -> (16.5403, -33.4425) construction
  line L64 (16.5403, -33.4425) -> (-9.9781, -33.4425) construction
  line L65 (-9.9781, -33.4425) -> (-9.9781, -25.3607) construction
  line L66 (-271.7189, -25.3359) -> (-321.7189, -25.3359) projected
  line L67 (-271.7189, -25.3359) -> (-221.7189, -25.3359) projected
  line L68 (-171.7189, -25.3359) -> (-221.7189, -25.3359) projected
  line L69 (-171.7189, -25.3359) -> (-121.7189, -25.3359) projected
  line L70 (-71.7189, -25.3359) -> (-121.7189, -25.3359) projected
  line L71 (-71.7189, -25.3359) -> (-21.7189, -25.3359) projected
  line L72 (28.2811, -25.3359) -> (-21.7189, -25.3359) projected
  line L73 (38.8877, 385.2707) -> (38.8877, -35.9425) projected
  line L74 (36.3877, 385.2707) -> (36.3877, -35.9425) construction
  line L75 (34.9933, -2.2119) -> (34.9933, 1.5401) construction
  line L76 (34.9933, 1.5401) -> (36.3877, 1.5401) construction
  line L77 (36.3877, 1.5401) -> (36.3877, -2.2119) construction
  line L78 (36.3877, -2.2119) -> (34.9933, -2.2119) construction
  line L79 (28.2811, 24.6641) -> (-21.7189, 24.6641) projected
  line L80 (28.2811, 24.6641) -> (28.2811, 74.6641) projected
  line L81 (-21.7189, 74.6641) -> (28.2811, 74.6641) projected
  line L82 (-21.7189, 24.6641) -> (-21.7189, 74.6641) projected
  line L83 (28.2811, 74.6641) -> (-21.7189, 74.6641) projected
  line L84 (28.2811, 124.6641) -> (28.2811, 74.6641) projected
  line L85 (-21.7189, 124.6641) -> (28.2811, 124.6641) projected
  line L86 (-21.7189, 74.6641) -> (-21.7189, 124.6641) projected
  line L87 (28.2811, 124.6641) -> (-21.7189, 124.6641) projected
  line L88 (28.2811, 124.6641) -> (28.2811, 174.6641) projected
  line L89 (-21.7189, 174.6641) -> (28.2811, 174.6641) projected
  line L90 (-21.7189, 124.6641) -> (-21.7189, 174.6641) projected
  line L91 (28.2811, 224.6641) -> (-21.7189, 224.6641) projected
  line L92 (28.2811, 224.6641) -> (28.2811, 274.6641) projected
  line L93 (-21.7189, 274.6641) -> (28.2811, 274.6641) projected
  line L94 (-21.7189, 224.6641) -> (-21.7189, 274.6641) projected
  line L95 (28.2811, 274.6641) -> (-21.7189, 274.6641) projected
  line L96 (28.2811, 324.6641) -> (28.2811, 274.6641) projected
  line L97 (-21.7189, 324.6641) -> (28.2811, 324.6641) projected
  line L98 (-21.7189, 274.6641) -> (-21.7189, 324.6641) projected
  line L99 (28.2811, 174.6641) -> (-21.7189, 174.6641) projected
  line L100 (28.2811, 224.6641) -> (28.2811, 174.6641) projected
  line L101 (-21.7189, 224.6641) -> (28.2811, 224.6641) projected
  line L102 (-21.7189, 174.6641) -> (-21.7189, 224.6641) projected
  line L103 (28.2811, 324.6641) -> (-21.7189, 324.6641) projected
  line L104 (28.2811, 324.6641) -> (28.2811, 374.6641) projected
  line L105 (28.2811, 374.6641) -> (-21.7189, 374.6641) projected
  line L106 (-21.7189, 324.6641) -> (-21.7189, 374.6641) projected
  line L107 (28.2811, 24.6641) -> (28.2811, -25.3359) projected
  line L108 (26.6749, 46.5018) -> (26.6749, 52.8264) construction
  line L109 (26.6749, 52.8264) -> (36.3877, 52.8264) construction
  line L110 (36.3877, 52.8264) -> (36.3877, 46.5018) construction
  line L111 (36.3877, 46.5018) -> (26.6749, 46.5018) construction
  line L112 (23.8996, 97.0416) -> (23.8996, 102.2866) construction
  line L113 (23.8996, 102.2866) -> (36.3877, 102.2866) construction
  line L114 (36.3877, 102.2866) -> (36.3877, 97.0416) construction
  line L115 (36.3877, 97.0416) -> (23.8996, 97.0416) construction
  line L116 (23.1503, 146.1674) -> (23.1503, 153.1608) construction
  line L117 (23.1503, 153.1608) -> (36.3877, 153.1608) construction
  line L118 (36.3877, 153.1608) -> (36.3877, 146.1674) construction
  line L119 (36.3877, 146.1674) -> (23.1503, 146.1674) construction
  line L120 (23.7336, 196.2518) -> (23.7336, 203.0765) construction
  line L121 (23.7336, 203.0765) -> (36.3877, 203.0765) construction
  line L122 (36.3877, 203.0765) -> (36.3877, 196.2518) construction
  line L123 (36.3877, 196.2518) -> (23.7336, 196.2518) construction
  line L124 (31.1324, 248.4972) -> (31.1324, 250.8311) construction
  line L125 (31.1324, 250.8311) -> (36.3877, 250.8311) construction
  line L126 (36.3877, 250.8311) -> (36.3877, 248.4972) construction
  line L127 (36.3877, 248.4972) -> (31.1324, 248.4972) construction
  line L128 (13.2122, 296.8205) -> (13.2122, 302.5077) construction
  line L129 (13.2122, 302.5077) -> (36.3877, 302.5077) construction
  line L130 (36.3877, 302.5077) -> (36.3877, 296.8205) construction
  line L131 (36.3877, 296.8205) -> (13.2122, 296.8205) construction
  line L132 (19.1838, 346.6783) -> (19.1838, 352.6499) construction
  line L133 (19.1838, 352.6499) -> (36.3877, 352.6499) construction
  line L134 (36.3877, 352.6499) -> (36.3877, 346.6783) construction
  line L135 (36.3877, 346.6783) -> (19.1838, 346.6783) construction
  line L136 (28.2811, 24.6641) -> (28.2811, 74.6641) projected
  line L137 (28.2811, 124.6641) -> (28.2811, 74.6641) projected
  line L138 (28.2811, 124.6641) -> (28.2811, 174.6641) projected
  line L139 (28.2811, 224.6641) -> (28.2811, 174.6641) projected
  line L140 (28.2811, 224.6641) -> (28.2811, 274.6641) projected
  line L141 (28.2811, 324.6641) -> (28.2811, 274.6641) projected
  line L142 (28.2811, 324.6641) -> (28.2811, 374.6641) projected
  line L143 (36.3877, 351.1511) -> (36.3877, 350.5191)
  line L144 (36.3877, 350.5191) -> (34.2483, 350.5191)
  spline S0 degree 2 poles (34.2483, 350.5191) (33.989, 350.5191) (33.5433, 350.4704) (33.4096, 350.3975) knots 0 0 0 1 2 2 2
  spline S1 degree 2 poles (33.4096, 350.3975) (33.2678, 350.3205) (33.13, 350.045) (33.13, 349.81) knots 0 0 0 1 2 2 2
  spline S2 degree 2 poles (33.13, 349.81) (33.13, 349.575) (33.3812, 349.0766) (33.5838, 348.8375) knots 0 0 0 1 2 2 2
  line L145 (33.5838, 348.8375) -> (36.3877, 348.8375)
  line L146 (36.3877, 348.8375) -> (36.3877, 348.2054)
  line L147 (36.3877, 348.2054) -> (31.1648, 348.2054)
  line L148 (31.1648, 348.2054) -> (31.1648, 348.8375)
  line L149 (31.1648, 348.8375) -> (33.053, 348.8375)
  spline S3 degree 2 poles (33.053, 348.8375) (32.7977, 349.1212) (32.5303, 349.6682) (32.5303, 349.9761) knots 0 0 0 1 2 2 2
  spline S4 degree 2 poles (32.5303, 349.9761) (32.5303, 350.5272) (33.2597, 351.1511) (33.9525, 351.1511) knots 0 0 0 1 2 2 2
  line L150 (33.9525, 351.1511) -> (36.3877, 351.1511)
  spline S5 degree 2 poles (35.5692, 298.3554) (35.5976, 298.4202) (35.6867, 298.6674) (35.7232, 298.8254) knots 0 0 0 1 2 2 2
  spline S6 degree 2 poles (35.7232, 298.8254) (35.7678, 298.9996) (35.8204, 299.2954) (35.8204, 299.4696) knots 0 0 0 1 2 2 2
  spline S7 degree 2 poles (35.8204, 299.4696) (35.8204, 299.7614) (35.6665, 300.1665) (35.5287, 300.28) knots 0 0 0 1 2 2 2
  spline S8 degree 2 poles (35.5287, 300.28) (35.3909, 300.3894) (35.0303, 300.4745) (34.7994, 300.4745) knots 0 0 0 1 2 2 2
  line L151 (34.7994, 300.4745) -> (34.4712, 300.4745)
  spline S9 degree 2 poles (34.4712, 300.4745) (34.694, 300.2192) (34.9047, 299.7289) (34.9047, 299.3602) knots 0 0 0 1 2 2 2
  spline S10 degree 2 poles (34.9047, 299.3602) (34.9047, 298.72) (33.9525, 297.9623) (33.0571, 297.9623) knots 0 0 0 1 2 2 2
  spline S11 degree 2 poles (33.0571, 297.9623) (32.5911, 297.9623) (31.8699, 298.2257) (31.6146, 298.4445) knots 0 0 0 1 2 2 2
  spline S12 degree 2 poles (31.6146, 298.4445) (31.3755, 298.6552) (31.1122, 299.2346) (31.1122, 299.5426) knots 0 0 0 1 2 2 2
  spline S13 degree 2 poles (31.1122, 299.5426) (31.1122, 299.8343) (31.2499, 300.2597) (31.3755, 300.4745) knots 0 0 0 1 2 2 2
  line L152 (31.3755, 300.4745) -> (31.2175, 300.511)
  line L153 (31.2175, 300.511) -> (31.2175, 301.1066)
  line L154 (31.2175, 301.1066) -> (34.5401, 301.1066)
  spline S14 degree 2 poles (34.5401, 301.1066) (35.4963, 301.1066) (36.3877, 300.2759) (36.3877, 299.421) knots 0 0 0 1 2 2 2
  spline S15 degree 2 poles (36.3877, 299.421) (36.3877, 299.1455) (36.2986, 298.5701) (36.2256, 298.3229) knots 0 0 0 1 2 2 2
  line L155 (36.2256, 298.3229) -> (35.5692, 298.3229)
  line L156 (35.5692, 298.3229) -> (35.5692, 298.3554)
  line L157 (33.9525, 300.4745) -> (31.8901, 300.4745)
  spline S16 degree 2 poles (31.8901, 300.4745) (31.7767, 300.2395) (31.6794, 299.8424) (31.6794, 299.6439) knots 0 0 0 1 2 2 2
  spline S17 degree 2 poles (31.6794, 299.6439) (31.6794, 299.1657) (32.3845, 298.6147) (33.0449, 298.6147) knots 0 0 0 1 2 2 2
  spline S18 degree 2 poles (33.0449, 298.6147) (33.6689, 298.6147) (34.3213, 299.032) (34.3213, 299.502) knots 0 0 0 1 2 2 2
  spline S19 degree 2 poles (34.3213, 299.502) (34.3213, 299.7492) (34.1268, 300.2678) (33.9525, 300.4745) knots 0 0 0 1 2 2 2
  line L158 (31.7726, 250.9283) -> (31.7726, 250.8959)
  spline S20 degree 2 poles (31.7726, 250.8959) (31.7402, 250.8108) (31.6835, 250.4947) (31.6835, 250.3691) knots 0 0 0 1 2 2 2
  spline S21 degree 2 poles (31.6835, 250.3691) (31.6835, 249.9721) (32.0401, 249.6317) (32.5101, 249.6317) knots 0 0 0 1 2 2 2
  line L159 (32.5101, 249.6317) -> (32.6357, 249.6317)
  line L160 (32.6357, 249.6317) -> (32.6357, 250.6771)
  line L161 (32.6357, 250.6771) -> (33.1584, 250.6771)
  line L162 (33.1584, 250.6771) -> (33.1584, 249.652)
  line L163 (33.1584, 249.652) -> (36.3877, 249.652)
  line L164 (36.3877, 249.652) -> (36.3877, 249.0199)
  line L165 (36.3877, 249.0199) -> (33.1584, 249.0199)
  line L166 (33.1584, 249.0199) -> (33.1584, 248.5944)
  line L167 (33.1584, 248.5944) -> (32.6357, 248.5944)
  line L168 (32.6357, 248.5944) -> (32.6357, 249.0199)
  line L169 (32.6357, 249.0199) -> (32.5101, 249.0199)
  spline S22 degree 2 poles (32.5101, 249.0199) (31.8375, 249.0199) (31.1324, 249.6722) (31.1324, 250.28) knots 0 0 0 1 2 2 2
  spline S23 degree 2 poles (31.1324, 250.28) (31.1324, 250.4542) (31.1689, 250.7905) (31.1932, 250.9283) knots 0 0 0 1 2 2 2
  line L170 (31.1932, 250.9283) -> (31.7726, 250.9283)
  spline S24 degree 2 poles (36.3877, 199.9417) (36.3877, 199.0422) (35.3788, 198.0535) (34.4469, 198.0535) knots 0 0 0 1 2 2 2
  spline S25 degree 2 poles (34.4469, 198.0535) (33.5311, 198.0535) (32.4452, 199.0138) (32.4452, 199.7877) knots 0 0 0 1 2 2 2
  spline S26 degree 2 poles (32.4452, 199.7877) (32.4452, 200.1362) (32.6478, 200.6751) (32.8626, 200.8736) knots 0 0 0 1 2 2 2
  spline S27 degree 2 poles (32.8626, 200.8736) (33.0773, 201.0762) (33.6973, 201.2909) (34.147, 201.2909) knots 0 0 0 1 2 2 2
  line L171 (34.147, 201.2909) -> (34.4914, 201.2909)
  line L172 (34.4914, 201.2909) -> (34.4914, 198.6937)
  spline S28 degree 2 poles (34.4914, 198.6937) (35.1438, 198.6937) (35.8366, 199.3501) (35.8366, 199.9336) knots 0 0 0 1 2 2 2
  spline S29 degree 2 poles (35.8366, 199.9336) (35.8366, 200.1402) (35.7435, 200.5413) (35.6705, 200.7034) knots 0 0 0 1 2 2 2
  spline S30 degree 2 poles (35.6705, 200.7034) (35.5895, 200.8736) (35.4477, 201.1086) (35.3828, 201.1856) knots 0 0 0 1 2 2 2
  line L173 (35.3828, 201.1856) -> (35.3828, 201.2221)
  line L174 (35.3828, 201.2221) -> (36.0717, 201.2221)
  spline S31 degree 2 poles (36.0717, 201.2221) (36.1162, 201.1127) (36.2459, 200.7804) (36.2824, 200.6507) knots 0 0 0 1 2 2 2
  spline S32 degree 2 poles (36.2824, 200.6507) (36.335, 200.4684) (36.3877, 200.1686) (36.3877, 199.9417) knots 0 0 0 1 2 2 2
  spline S33 degree 2 poles (34.0093, 200.6751) (33.754, 200.667) (33.3812, 200.5616) (33.2556, 200.4603) knots 0 0 0 1 2 2 2
  spline S34 degree 2 poles (33.2556, 200.4603) (33.1138, 200.3509) (32.9639, 200.0065) (32.9639, 199.7512) knots 0 0 0 1 2 2 2
  spline S35 degree 2 poles (32.9639, 199.7512) (32.9639, 199.5) (33.1138, 199.1475) (33.2597, 199.0016) knots 0 0 0 1 2 2 2
  spline S36 degree 2 poles (33.2597, 199.0016) (33.4096, 198.8598) (33.7702, 198.714) (34.0093, 198.6937) knots 0 0 0 1 2 2 2
  line L175 (34.0093, 198.6937) -> (34.0093, 200.6751)
  line L176 (36.2824, 151.1066) -> (36.2824, 150.4745)
  line L177 (36.2824, 150.4745) -> (35.9015, 150.4745)
  spline S37 degree 2 poles (35.9015, 150.4745) (36.023, 150.3286) (36.1851, 150.1139) (36.254, 149.968) knots 0 0 0 1 2 2 2
  spline S38 degree 2 poles (36.254, 149.968) (36.3188, 149.8343) (36.3877, 149.5466) (36.3877, 149.3562) knots 0 0 0 1 2 2 2
  spline S39 degree 2 poles (36.3877, 149.3562) (36.3877, 149.0482) (36.1324, 148.5296) (35.8853, 148.3473) knots 0 0 0 1 2 2 2
  spline S40 degree 2 poles (35.8853, 148.3473) (35.6381, 148.1649) (34.9088, 147.9623) (34.4347, 147.9623) knots 0 0 0 1 2 2 2
  spline S41 degree 2 poles (34.4347, 147.9623) (33.9404, 147.9623) (33.2191, 148.2176) (32.9477, 148.4405) knots 0 0 0 1 2 2 2
  spline S42 degree 2 poles (32.9477, 148.4405) (32.7046, 148.6471) (32.425, 149.2265) (32.425, 149.5466) knots 0 0 0 1 2 2 2
  spline S43 degree 2 poles (32.425, 149.5466) (32.425, 149.8262) (32.5506, 150.2435) (32.6802, 150.4745) knots 0 0 0 1 2 2 2
  line L178 (32.6802, 150.4745) -> (31.0595, 150.4745)
  line L179 (31.0595, 150.4745) -> (31.0595, 151.1066)
  line L180 (31.0595, 151.1066) -> (36.2824, 151.1066)
  line L181 (35.3707, 150.4745) -> (33.2029, 150.4745)
  spline S44 degree 2 poles (33.2029, 150.4745) (33.0895, 150.2395) (33.0044, 149.8667) (33.0044, 149.652) knots 0 0 0 1 2 2 2
  spline S45 degree 2 poles (33.0044, 149.652) (33.0044, 149.1657) (33.7337, 148.6147) (34.4225, 148.6147) knots 0 0 0 1 2 2 2
  spline S46 degree 2 poles (34.4225, 148.6147) (35.0871, 148.6147) (35.788, 149.0361) (35.788, 149.502) knots 0 0 0 1 2 2 2